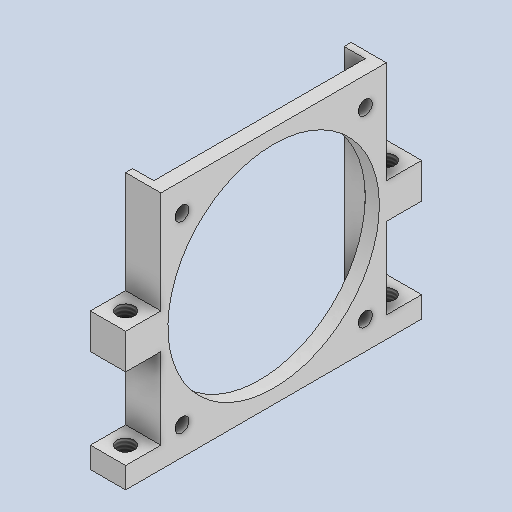
# Autodesk Inventor part: Camera holder
Saved by Autodesk Inventor 2023 (Build 270158000, 158)
## iProperties
Created: 2023-04-08
Part Number: Camera holder
Material: Generic
Document SubType Name: Modeling
Designer: ASARe-DAQ-PC
Density: 1 g/cm^3
Appearance: Default
Author: ASARe-DAQ-PC
Autodesk Inventor part; units mm, degrees
ref_plane "YZ Plane" through (0, 0, 0) normal (1, 0, 0) x (0, 1, 0)
ref_plane "XZ Plane" through (0, 0, 0) normal (0, 1, 0) x (-1, 0, 0)
ref_plane "XY Plane" through (0, 0, 0) normal (0, 0, 1) x (1, 0, 0)
sketch "Sketch1" plane through (0, 0, 0) normal (1, 0, 0) x (0, 1, 0)
  circle A0 centre (0, 0) radius 15
  line L0 (15, 15) -> (-15, 15)
  line L1 (-15, 15) -> (-15, -15) construction
  line L2 (-15, -15) -> (15, -15)
  line L3 (15, -15) -> (15, 15) construction
  line L4 (15, 15) -> (-15, -15) construction
  line L5 (-15, 15) -> (15, -15) construction
  line L6 (17, 21) -> (-17, 21)
  line L7 (-17, 21) -> (-17, -21)
  line L8 (-17, -21) -> (17, -21)
  line L9 (17, -21) -> (17, 21)
  line L10 (17, 21) -> (-17, -21) construction
  line L11 (-17, 21) -> (17, -21) construction
  circle A1 centre (13, -13) radius 1
  circle A2 centre (13, 13) radius 1
  circle A3 centre (-13, -13) radius 1
  circle A4 centre (-13, 13) radius 1
  line L12 (17, -15) -> (15, -15)
  line L13 (-15, -15) -> (-17, -15)
  line L14 (17, 15) -> (15, 15)
  line L15 (-15, 15) -> (-17, 15)
  point P0 (0, -15)
  point P1 (0, 15)
  dimension "d0" = 30
  dimension "d1" = 42
  dimension "d2" = 34
  dimension "d10" = 2
  dimension "d11" = 2
  dimension "d14" = 26
  dimension "d17" = 26
  constraints: 32 end point, 7 point on line, 5 centre point, 5 parallel, 4 midpoint, 3 horizontal, 3 perpendicular, 2 tangent, 1 coincident, 1 vertical, 6 other
  measures "d0" diameter of A0
  measures "d1" distance of L8.end L6.start
  measures "d2" distance of L6.start L6.end
  measures "d10" diameter of A1
  measures "d11" horizontal distance of L2.end A1.centre
  measures "d14" distance of A1.centre A2.centre
  measures "d17" distance of A1.centre A3.centre
sketch "Sketch2" plane through (0, 0, 0) normal (0, 1, 0) x (-1, 0, 0)
  line L0 (190, 50) -> (-10, 50)
  line L1 (-10, 50) -> (-10, -50)
  line L2 (-10, -50) -> (190, -50)
  line L3 (190, -50) -> (190, 50)
  point P0 (0, 0)
  point P1 (-10, 0)
  dimension "d3" = 200
  dimension "d4" = 100
  dimension "d5" = 10
  constraints: 8 end point, 2 parallel, 1 horizontal, 1 horizontal alignment, 1 midpoint, 1 perpendicular
  measures "d3" distance of L1.end L2.end
  measures "d4" distance of L0.end L1.end
  measures "d5" distance from line of L1 point (0, 0)
extrude "Extrusion1" add sketch "Sketch1" along normal blind 5 contours A0 | A0 L0 L14 L9 L12 L2 | L0 L15 L7 L6 L9 L14 | A0 L2 L13 L7 L15 L0 | L2 L12 L9 L8 L7 L13 | A1 | A2 | A3 | A4
extrude "Extrusion4" cut sketch "Sketch1" along normal blind 3 contours A0 L0 L14 L9 L12 L2 | A0 L2 L13 L7 L15 L0
extrude "Extrusion3" cut sketch "Sketch1" along normal blind 5 contours A0 | A1 | A2 | A3 | A4
sketch "Sketch3" plane through (0, -17, 21) normal (0, 0, 1) x (1, 0, 0)
  line L0 (0, 34) -> (0, 0) projected
  line L1 (0, 0) -> (5, 0) projected
  line L2 (5, 34) -> (5, 0) projected
  line L3 (0, 34) -> (5, 34) projected
  line L4 (0, 0) -> (0, 34) projected
  line L5 (5, 0) -> (5, 34) projected
  line L6 (0, 14.5) -> (5, 14.5)
  line L7 (5, 14.5) -> (5, 3)
  line L8 (5, 3) -> (0, 3)
  line L9 (0, 3) -> (0, 14.5)
  line L10 (0, 34) -> (5, 34)
  line L11 (5, 34) -> (5, 19.5)
  line L12 (5, 19.5) -> (0, 19.5)
  line L13 (0, 19.5) -> (0, 34)
  point P0 (0, 17)
  point P1 (0, 17)
  point P2 (0, 3)
  point P3 (5, 3)
  point P4 (0, 19.5)
  dimension "d26" = 3
  dimension "d27" = 5
  dimension "d29" = 2.5
  constraints: 16 end point, 5 point on line, 4 parallel, 2 horizontal, 2 perpendicular, 1 midpoint
  measures "d26" distance between parallel lines of L1 L8
  measures "d27" distance between parallel lines of L6 L12
  measures "d29" distance from line of point (0, 17) L12
extrude "Extrusion5" cut sketch "Sketch3" against normal blind 5 contours L3 L2 L12 L0 | L6 L2 L8 L0
mirror "Mirror1" about plane through (0, 0, 0) normal (0, 0, 1) of "Extrusion5"
sketch "Sketch4" plane through (0, -17, -21) normal (0, -1, 0) x (1, 0, 0)
  line L0 (5, 42) -> (5, 0) projected
  line L1 (0, 0) -> (5, 0) projected
  line L2 (0, 42) -> (5, 42) projected
  point P0 (0, 21)
  point P1 (2.5, 39.5)
  point P2 (2.5, 2.5)
  dimension "d39" = 2.5
  dimension "d40" = 2.5
  dimension "d41" = 2.5
  dimension "d42" = 2.5
  measures "d39" distance from line of L0 point (2.5, 2.5)
  measures "d40" distance from line of L1 point (2.5, 2.5)
  measures "d41" distance from line of L0 point (2.5, 39.5)
  measures "d42" distance from line of L2 point (2.5, 39.5)
hole "Hole1" at (2.5, -17, 18.5) at (2.5, -17, -18.5) direction (0, 1, 0) diameter 2.459 end through all thread size "M3x0.5" class "6H" standard "ISO Metric profile"
body "Solid1"
body "Solid3"
body "Solid4"
